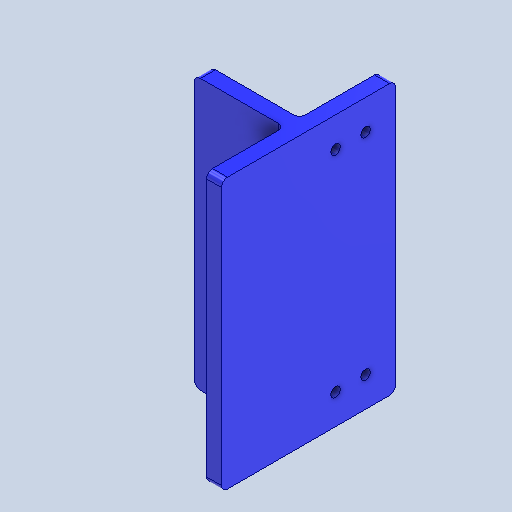
# Autodesk Inventor part: dribl-v3-3DP-2
Saved by Autodesk Inventor 2025.2 (Build 292293000, 293)
## iProperties
Created: 2025-04-18
Part Number: dribl-v3-3DP-2
Material: ABS プラスチック
Document SubType Name: Modeling
Designer: haruy
Density: 1.06 g/cm^3
Appearance: 青 - 壁塗料 - 光沢
Author: haruy
Autodesk Inventor part; units mm, degrees
ref_plane "YZ Plane" through (0, 0, 0) normal (1, 0, 0) x (0, 1, 0)
ref_plane "XZ Plane" through (0, 0, 0) normal (0, 1, 0) x (-1, 0, 0)
ref_plane "XY Plane" through (0, 0, 0) normal (0, 0, 1) x (1, 0, 0)
sketch "スケッチ1" plane through (0, 0, 0) normal (1, 0, 0) x (0, 1, 0)
  line L0 (-10.8312, -155.4782) -> (79.1688, -155.4782)
  line L1 (79.1688, -155.4782) -> (79.1688, -129.4782)
  line L2 (79.1688, -129.4782) -> (-10.8312, -129.4782)
  line L3 (-10.8312, -129.4782) -> (-10.8312, -155.4782)
  line L4 (-10.8312, -187.4782) -> (-10.8312, 372.5218)
  line L5 (79.1688, 372.5218) -> (79.1688, -187.4782)
  line L6 (-10.8312, -187.4782) -> (79.1688, -187.4782)
  line L7 (79.1688, -187.4782) -> (79.1688, -160.4782)
  line L8 (79.1688, -160.4782) -> (-10.8312, -160.4782)
  line L9 (-10.8312, -160.4782) -> (-10.8312, -187.4782)
  circle A0 centre (-0.8312, -167.4782) radius 1.6
  line L10 (-10.8312, -160.4782) -> (79.1688, -160.4782)
  line L11 (79.1688, -160.4782) -> (79.1688, -129.4782)
  line L12 (79.1688, -129.4782) -> (-10.8312, -129.4782)
  line L13 (-10.8312, -129.4782) -> (-10.8312, -160.4782)
  circle A1 centre (-0.8312, -167.4782) radius 1.6
  circle A2 centre (-0.8312, -177.4782) radius 1.6
  circle A3 centre (-0.8312, -177.4782) radius 1.6
  circle A4 centre (69.1688, -167.4782) radius 1.6
  circle A5 centre (69.1688, -167.4782) radius 1.6
  circle A6 centre (69.1688, -177.4782) radius 1.6
  circle A7 centre (69.1688, -177.4782) radius 1.6
  point P0 (0, 0)
  point P1 (-65.8312, -380.4782)
  dimension "d0" = 90
  dimension "d1" = 26
  dimension "d2" = 7
  dimension "d3" = 5
  dimension "d4" = 0
  dimension "d5" = 3.2
  dimension "d6" = 3.2
  dimension "d7" = 3.2
  dimension "d8" = 3.2
  constraints: 28 end point, 8 centre point, 6 parallel, 4 coincident, 3 horizontal, 3 perpendicular, 1 point on line
  measures "d0" distance of L2.end L1.end
  measures "d1" distance of L1.end L0.end
  measures "d2" distance from line of A0.centre L8
  measures "d3" distance between parallel lines of L0 L8
  measures "d4" distance between parallel lines of L5 L1
  measures "d5" diameter of A1
  measures "d6" diameter of A3
  measures "d7" diameter of A5
  measures "d8" diameter of A7
extrude "押し出し1" add sketch "スケッチ1" along normal blind 5
extrude "押し出し2" add sketch "スケッチ1" against normal blind 30 contours L0 L5 L8 L4
sketch "スケッチ2" plane through (0, -10.8312, -160.4782) normal (0, 0, -1) x (-1, 0, 0)
  line L0 (30, 90) -> (30, 0) projected
  line L1 (30, 45) -> (0, 45)
  line L2 (0, 0) -> (30, 0) projected
  line L3 (17.5, 0) -> (17.5, 90)
  line L4 (0, 90) -> (30, 90) projected
  circle A0 centre (17.5, 22.5) radius 1.6
  circle A1 centre (17.5, 67.5) radius 1.6
  point P0 (0, 10.8312)
  point P1 (15, 45)
  dimension "d13" = 12.5
  dimension "d14" = 3.2
  dimension "d15" = 3.2
  dimension "d16" = 22.5
  dimension "d17" = 22.5
  constraints: 4 end point, 4 point on line, 2 centre point, 2 midpoint, 1 horizontal, 1 vertical
  measures "d13" distance between parallel lines of L0 L3
  measures "d14" diameter of A0
  measures "d15" diameter of A1
  measures "d16" vertical distance of A0.centre point (15, 45)
  measures "d17" distance from line of A1.centre L1
hole "穴1" at (-17.5, 11.6688, -160.4782) at (-17.5, 56.6688, -160.4782) direction (0, 0, 1) diameter 3.2 end through all
fillet "フィレット1" radius 2 8 edges at (0, 34.1688, -160.4782) (-30, -10.8312, -157.9782) (-30, 79.1688, -157.9782) (0, 34.1688, -155.4782) (2.5, -10.8312, -187.4782) (2.5, 79.1688, -187.4782) (2.5, 79.1688, -129.4782) (2.5, -10.8312, -129.4782)
equation "\"d17\" = d16"
